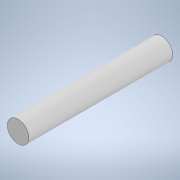
# Autodesk Inventor part: Servo motor support rods
Saved by Autodesk Inventor 2021 (Build 250183000, 183)
## iProperties
Created: 2021-06-28
Part Number: Servo motor support rods
Material: Generic
Document SubType Name: Modeling
Designer: Michael Swaminathan
Density: 1 g/cm^3
Appearance: Default
Author: Michael Swaminathan
Autodesk Inventor part; units mm, degrees
ref_plane "YZ Plane" through (0, 0, 0) normal (1, 0, 0) x (0, 1, 0)
ref_plane "XZ Plane" through (0, 0, 0) normal (0, 1, 0) x (-1, 0, 0)
ref_plane "XY Plane" through (0, 0, 0) normal (0, 0, 1) x (1, 0, 0)
sketch "Sketch1" plane through (0, 0, 0) normal (0, 0, 1) x (1, 0, 0)
  circle A0 centre (-20.6655, 9.3226) radius 1.5
  point P0 (0, 0)
  dimension "d0" = 3
  dimension "d0" = 3
  constraints: 1 centre point
  measures "d0" diameter of A0
extrude "Extrusion1" add sketch "Sketch1" along normal blind 20
body "Solid1"
